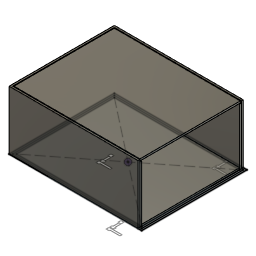
do not disturb v1 (Autodesk Fusion 360 design; units mm, degrees)
Autodesk Fusion 360 part; units mm, degrees
sketch "Sketch1" plane through (0, 0, 0) normal (0, 1, 0) x (1, 0, 0) in component "Bottom"
  line L0 (27.5, 21.5) -> (-27.5, 21.5)
  line L1 (-27.5, 21.5) -> (-27.5, -21.5)
  line L2 (-27.5, -21.5) -> (27.5, -21.5)
  line L3 (27.5, -21.5) -> (27.5, 21.5)
  line L4 (27.5, 21.5) -> (-27.5, -21.5) construction
  line L5 (-27.5, 21.5) -> (27.5, -21.5) construction
  line L6 (-28.3, 22.3) -> (-28.3, -22.3)
  line L7 (-28.3, -22.3) -> (28.3, -22.3)
  line L8 (28.3, -22.3) -> (28.3, 22.3)
  line L9 (28.3, 22.3) -> (-28.3, 22.3)
  line L10 (-29.1, 23.1) -> (-29.1, -23.1)
  line L11 (-29.1, -23.1) -> (29.1, -23.1)
  line L12 (29.1, -23.1) -> (29.1, 23.1)
  line L13 (29.1, 23.1) -> (-29.1, 23.1)
  line L14 (27.5, 21.5) -> (27.5, 23.1)
  line L15 (27.5, -21.5) -> (27.5, -23.1)
  dimension "d1" = 55
  dimension "d2" = 43
  dimension "d8" = 0.8
  dimension "d9" = 1.6
  constraint horizontal L0
  constraint perpendicular L0 L1
  constraint parallel L0 L2
  constraint parallel L1 L3
  constraint coincident L4 origin
  constraint coincident L5 origin
  constraint coincident L13 L14.end
  constraint perpendicular L13 L14
  constraint coincident L11 L15.end
  constraint perpendicular L11 L15
  measures "d1" distance of L1.end L2.end
  measures "d2" distance of L0.end L1.end
extrude "Extrude2" add sketch "Sketch1" along normal blind 25 contours L0 L1 L2 L6 L7 L9 L14 L15 makes body 1 in component "Bottom"
extrude "Extrude1" add sketch "Sketch1" along normal blind 0.8 separate body contours L0 L1 L2 L3 makes body 2 in component "Bottom"
extrude "Extrude3" add sketch "Sketch1" along normal blind 25.8 separate body contours L6 L7 L9 L10 L11 L13 L14 L15 makes body 3 in component "Bottom"
sketch "Sketch2" plane through (0, 0, 0) normal (0, 1, 0) x (1, 0, 0) in component "Bottom"
sketch "Sketch2 (2)" plane through (0, 25, 0) normal (0, 1, 0) x (-1, 0, 0) in component "Top"
  line L0 (-27.5, -21.5) -> (-27.5, -22.3)
  line L1 (-27.5, -22.3) -> (28.3, -22.3)
  line L2 (28.3, -22.3) -> (28.3, 22.3)
  line L3 (28.3, 22.3) -> (-27.5, 22.3)
  line L4 (-27.5, 22.3) -> (-27.5, 21.5)
  line L5 (-27.5, 21.5) -> (27.5, 21.5)
  line L6 (27.5, 21.5) -> (27.5, -21.5)
  line L7 (27.5, -21.5) -> (-27.5, -21.5)
  line L8 (28.3, -22.3) -> (-27.5, -22.3)
  line L9 (-27.5, -22.3) -> (-27.5, 22.3)
  line L10 (-27.5, 22.3) -> (28.3, 22.3)
  line L11 (28.3, 22.3) -> (28.3, -22.3)
  line L12 (-27.25, 22.05) -> (28.05, 22.05)
  line L13 (28.05, 22.05) -> (28.05, -22.05)
  line L14 (28.05, -22.05) -> (-27.25, -22.05)
  line L15 (-27.25, -22.05) -> (-27.25, 22.05)
  dimension "d18" = 0.25
  constraint horizontal L8
  constraint vertical L9
  constraint horizontal L10
  constraint vertical L11
  constraint coincident L3.end L4.start
  constraint coincident L1.end L2.start
extrude "Extrude1'" add sketch "Sketch2 (2)" along normal blind 0.8 separate body contours L5 L6 L7 L15 | L5 L6 L7 L12 L13 L14 L15 makes body 4 in component "Top"
component "Top" placed x (1, 0, 0) y (0, 1, 0) z (0, 0, 1) at (0, 0, 0)
component "Bottom" placed x (1, 0, 0) y (0, 1, 0) z (0, 0, 1) at (0, 0, 0)
equation "d1 = Length"
equation "d2 = Width"
equation "Width = 43 mm"
equation "Length = 55 mm"
equation "Height = 80 mm"
equation "InnerWall = 0.8 mm"
equation "OuterWall = 0.8 mm"
equation "d8 = InnerWall"
equation "d9 = InnerWall + OuterWall"
equation "d10 = InnerWall"
equation "InnerWallHeight = 25 mm"
equation "OuterWallheight = 30 mm"
equation "d14 = InnerWallHeight"
equation "d16 = InnerWallHeight + InnerWall"
equation "d19 = InnerWall"
